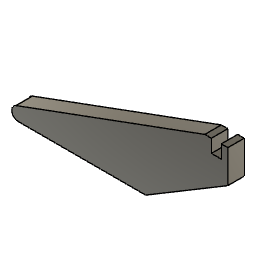
holder v2 (Autodesk Fusion 360 design; units mm, degrees)
Autodesk Fusion 360 part; units mm, degrees
sketch "Sketch1" plane through (0, 0, 0) normal (0, 1, 0) x (1, 0, 0)
  line L0 (0, 0) -> (50, 0)
  line L1 (50, 0) -> (75, -15)
  line L2 (75, -15) -> (75, -25)
  line L3 (75, -25) -> (68, -25)
  line L4 (68, -25) -> (0, 0)
  line L5 (70, -25) -> (73, -25)
  line L6 (73, -25) -> (73, -21)
  line L7 (73, -21) -> (70, -21)
  line L8 (70, -21) -> (70, -25)
  dimension "d1" = 50
  dimension "d3" = 15
  dimension "d4" = 25
  dimension "d7" = 7
  dimension "d8" = 3
  dimension "d9" = 4
  constraint coincident L0.start L4.end
  constraint horizontal L0
  constraint vertical L2
  constraint perpendicular L2 L3
  constraint horizontal L5
  constraint vertical L6
  constraint horizontal L7
  constraint vertical L8
  constraint coincident L3 L5.start
  measures "d1" distance of L0.start L0.end
  measures "d3" vertical distance of L0.end L1.end
  measures "d4" vertical distance of L3.end L0.start
  measures "d7" distance of L2.end L3.end
  measures "d8" distance of L5.start L5.end
  measures "d9" distance of L5.end L6.end
extrude "Extrude1" add sketch "Sketch1" along normal blind 5 contours L0 L1 L2 L3 L4 L6 L7 L8
fillet "Fillet1" radius 2 1 edges at (0, 2.5, 0)
